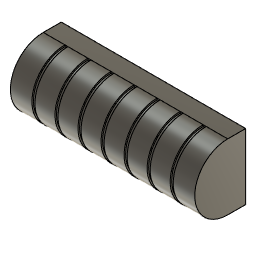
Front Greeblie SM (Autodesk Fusion 360 design; units mm, degrees)
Autodesk Fusion 360 part; units mm, degrees
sketch "Sketch1" plane through (0, 0, 0) normal (1, 0, 0) x (0, 1, 0)
  circle A0 centre (0, 0) radius 2.75
  line L0 (0, 0) -> (0, 2.75) construction
  line L1 (0, 0) -> (0, -2.75) construction
  line L2 (0, 2.75) -> (1.5, 2.75)
  line L3 (1.5, 2.75) -> (1.5, -2.75)
  line L4 (1.5, -2.75) -> (0, -2.75)
  line L5 (0, -2.75) -> (0, 2.75)
  dimension "d1" = 5.5
  dimension "d42" = 1.5
  constraint coincident A0.centre L0.start
  constraint coincident A0 L0.end
  constraint vertical L0
  constraint coincident A0 L1.end
  constraint parallel L0 L1
  constraint horizontal L2
  constraint vertical L3
  constraint horizontal L4
  constraint vertical L5
  measures "d1" diameter of A0
  measures "d42" distance of L0.end L2.end
extrude "Extrude1" add sketch "Sketch1" along normal mid plane 15.4 contours A0 L5 | A0 L3 L5 | A0 L3
ref_plane "WorkPlane1" through (-7.5, 0, 0) normal (-1, 0, 0) x (0, -1, 0)
ref_plane "WorkPlane2" through (0, 0, 0) normal (1, 0, 0) x (0, 1, 0)
ref_plane "WorkPlane3" through (3.85, 0, 0) normal (1, 0, 0) x (0, 1, 0)
ref_plane "WorkPlane4" through (5.775, 0, 0) normal (1, 0, 0) x (0, 1, 0)
ref_plane "WorkPlane5" through (1.925, 0, 0) normal (1, 0, 0) x (0, 1, 0)
ref_plane "WorkPlane6" through (-3.85, 0, 0) normal (-1, 0, 0) x (0, -1, 0)
ref_plane "WorkPlane7" through (-5.775, 0, 0) normal (-1, 0, 0) x (0, -1, 0)
ref_plane "WorkPlane8" through (-1.925, 0, 0) normal (-1, 0, 0) x (0, -1, 0)
sketch "Sketch3" plane through (0, 0, 0) normal (1, 0, 0) x (0, 1, 0)
  circle A0 centre (0, 0) radius 2.75
  circle A1 centre (0, 0) radius 2.625
  dimension "d12" = 5.5
  dimension "d13" = 5.25
  constraint coincident A0.centre A1.centre
  measures "d12" diameter of A0
  measures "d13" diameter of A1
extrude "Extrude2" cut sketch "Sketch3" along normal mid plane 0.25
sketch "Sketch4" plane through (-7.5, 0, 0) normal (-1, 0, 0) x (0, 1, 0)
  circle A0 centre (0, 0) radius 2.75
  circle A1 centre (0, 0) radius 2.625
  dimension "d16" = 5.5
  dimension "d17" = 5.25
  constraint coincident A0.centre A1.centre
  constraint concentric A0 A1
  measures "d16" diameter of A0
  measures "d17" diameter of A1
sketch "Sketch5" plane through (-1.925, 0, 0) normal (-1, 0, 0) x (0, 1, 0)
  circle A0 centre (0, 0) radius 2.75
  circle A1 centre (0, 0) radius 2.625
  dimension "d18" = 5.5
  dimension "d19" = 5.25
  constraint coincident A0.centre A1.centre
  constraint concentric A0 A1
  measures "d18" diameter of A0
  measures "d19" diameter of A1
extrude "Extrude3" cut sketch "Sketch5" along normal mid plane 0.25
sketch "Sketch6" plane through (-3.85, 0, 0) normal (-1, 0, 0) x (0, 1, 0)
  circle A0 centre (0, 0) radius 2.75
  circle A1 centre (0, 0) radius 2.625
  dimension "d22" = 5.5
  dimension "d23" = 5.25
  constraint coincident A0.centre A1.centre
  measures "d22" diameter of A0
  measures "d23" diameter of A1
extrude "Extrude4" cut sketch "Sketch6" along normal mid plane 0.25
sketch "Sketch7" plane through (-5.775, 0, 0) normal (-1, 0, 0) x (0, 1, 0)
  circle A0 centre (0, 0) radius 2.75
  circle A1 centre (0, 0) radius 2.625
  dimension "d26" = 5.5
  dimension "d27" = 5.25
  constraint coincident A0.centre A1.centre
  constraint concentric A0 A1
  measures "d26" diameter of A0
  measures "d27" diameter of A1
extrude "Extrude5" cut sketch "Sketch7" along normal mid plane 0.25
sketch "Sketch8" plane through (1.925, 0, 0) normal (1, 0, 0) x (0, 1, 0)
  circle A0 centre (0, 0) radius 2.75
  circle A1 centre (0, 0) radius 2.625
  dimension "d30" = 5.5
  dimension "d31" = 5.25
  constraint coincident A0.centre A1.centre
  measures "d30" diameter of A0
  measures "d31" diameter of A1
extrude "Extrude6" cut sketch "Sketch8" along normal mid plane 0.25
sketch "Sketch9" plane through (3.85, 0, 0) normal (1, 0, 0) x (0, 1, 0)
  circle A0 centre (0, 0) radius 2.75
  circle A1 centre (0, 0) radius 2.625
  dimension "d34" = 5.5
  dimension "d35" = 5.25
  constraint coincident A0.centre A1.centre
  constraint concentric A0 A1
  measures "d34" diameter of A0
  measures "d35" diameter of A1
extrude "Extrude7" cut sketch "Sketch9" along normal mid plane 0.25
sketch "Sketch10" plane through (5.775, 0, 0) normal (1, 0, 0) x (0, 1, 0)
  circle A0 centre (0, 0) radius 2.75
  circle A1 centre (0, 0) radius 2.625
  dimension "d38" = 5.5
  dimension "d39" = 5.25
  constraint coincident A0.centre A1.centre
  constraint concentric A0 A1
  measures "d38" diameter of A0
  measures "d39" diameter of A1
extrude "Extrude8" cut sketch "Sketch10" along normal mid plane 0.25
extrude "Extrude9" add sketch "Sketch1" along normal mid plane 15.4 contours A0 L2 L3 | A0 L3 L5 | A0 L3 L4
extrude "Extrude10" cut sketch "Sketch1" along normal mid plane 20 contours A0 L3
